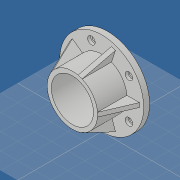
# Autodesk Inventor part: Zyklon_Flansch
Saved by Autodesk Inventor 2019 (Build 230136000, 136)
## iProperties
Created: 2020-08-01
Part Number: Zyklon_Flansch
Material: Generisch
Document SubType Name: Modeling
Designer: Stefan
Mass: 75.8697 g
Surface Area: 303.384 cm^2
Volume: 75.8697 cm^3
Density: 1 g/cm^3
Appearance: Vorgabe
Author: Stefan
Autodesk Inventor part; units mm, degrees
ref_plane "YZ Plane" through (0, 0, 0) normal (1, 0, 0) x (0, 1, 0)
ref_plane "XZ Plane" through (0, 0, 0) normal (0, 1, 0) x (-1, 0, 0)
ref_plane "XY Plane" through (0, 0, 0) normal (0, 0, 1) x (1, 0, 0)
sketch "Skizze1" plane through (0, 0, 0) normal (0, 0, 1) x (1, 0, 0)
  circle A0 centre (0, 0) radius 25.1
  circle A1 centre (0, 0) radius 50
  circle A2 centre (0, 0) radius 30
  dimension "d0" = 50.2
  dimension "d1" = 100
  dimension "d2" = 60
  constraints: 3 centre point, 3 coincident
  measures "d0" diameter of A0
  measures "d1" diameter of A1
  measures "d2" diameter of A2
extrude "Extrusion1" add sketch "Skizze1" against normal blind 7 contours A1 | A2
extrude "Extrusion2" add sketch "Skizze1" along normal blind 35 contours A2
sketch "Skizze2" plane through (0, 0, 0) normal (0, 1, 0) x (-1, 0, 0)
  line L0 (50, 0) -> (50, -7) projected
  line L1 (50, -7) -> (25.1, -7) projected
  line L2 (25.1, -7) -> (25.1, 35) projected
  line L3 (25.1, 35) -> (30, 35) projected
  line L4 (30, 35) -> (30, 0) projected
  line L5 (30, 0) -> (50, 0) projected
  line L6 (-50, -7) -> (-50, 0) projected
  line L7 (-50, 0) -> (-30, 0) projected
  line L8 (-30, 0) -> (-30, 35) projected
  line L9 (-30, 35) -> (-25.1, 35) projected
  line L10 (-25.1, 35) -> (-25.1, -7) projected
  line L11 (-25.1, -7) -> (-50, -7) projected
  line L12 (-30, 35) -> (-45, 0)
  line L13 (-30, 35) -> (-30, 0)
  line L14 (-30, 0) -> (-45, 0)
  line L15 (-25.1, 5) -> (-30, 5)
  line L16 (-30, 5) -> (-30, 35)
  line L17 (-30, 35) -> (-25.1, 35)
  line L18 (-25.1, 35) -> (-25.1, 5)
  line L19 (0, -12) -> (0, 37) projected
  point P0 (0, 0)
  dimension "d7" = 5
  constraints: 14 end point, 3 equal length, 2 perpendicular, 2 point on line, 1 horizontal
  measures "d7" distance from line of L6 L12.end
extrude "Extrusion3" add sketch "Skizze2" along normal mid plane 5 contours L12 L8 L7 | L15 L8 L9 L10
pattern_circular "Runde Anordnung1" count 5 over 360 about axis through (0, 0, -10) along (0, 0, 1) of "Extrusion3"
sketch "Skizze3" plane through (0, 0, 0) normal (0, 0, 1) x (1, 0, 0)
  arc A0 (9.2705, -28.5317) -> (30, 0) centre (0, 0) ccw projected
  circle A1 centre (0, 0) radius 40 construction
  point P0 (11.6159, -27.6599)
  point P1 (29.8957, -2.5)
  point P2 (-40, 0)
  dimension "d14" = 80
  constraints: 1 coincident, 1 horizontal alignment, 2 other
hole "Bohrung1" at (-40, 0, 0) direction (0, 0, -1) diameter 5.5 end through all counterbore diameter 9 counterbore depth 3.5 clearance for "Zylinderschraube mit Schlitz DIN 84" size "M5" standard "DIN"
pattern_circular "Runde Anordnung2" count 5 over 360 about axis through (0, 0, -10) along (0, 0, 1) of "Bohrung1"
equation "\"d0\" = ht_diameter + 2 * gap_fit"
equation "\"kg_thickness\" = 4.9"
equation "\"ht_thickness\" = 1.9"
equation "\"case_thickness\" = 18"
equation "\"gap_fit\" = 0.1"
equation "\"gap_slide\" = 0.2"
equation "\"gap_air\" = 1"
equation "\"bore_diameter\" = 73"
equation "\"mdf_thickness\" = 6"
equation "\"tape_thickness\" = 3"
equation "\"tape_width\" = 15"
equation "\"inner_thickness\" = 15"
equation "\"inner_depth\" = 255"
equation "\"ht_diameter\" = 50"
